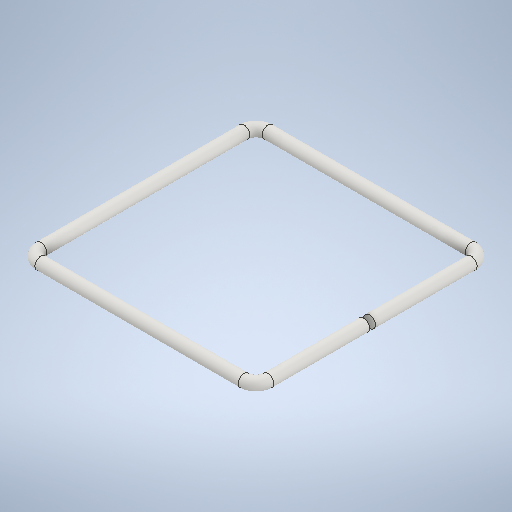
# Autodesk Inventor part: Ring_Of_Rebar
Saved by Autodesk Inventor 2025.1 (Build 291241020, 241B)
## iProperties
Created: 2024-09-07
Part Number: Ring_Of_Rebar
Material: Steel
Document SubType Name: Modeling
Designer: Tom
Density: 7.85 g/cm^3
Appearance: Steel
Author: Tom
Autodesk Inventor part; units mm, degrees
ref_plane "YZ Plane" through (0, 0, 0) normal (1, 0, 0) x (0, 1, 0)
ref_plane "XZ Plane" through (0, 0, 0) normal (0, 1, 0) x (-1, 0, 0)
ref_plane "XY Plane" through (0, 0, 0) normal (0, 0, 1) x (1, 0, 0)
sketch "Sketch1" plane through (0, 0, 0) normal (0, 0, 1) x (1, 0, 0)
  circle A0 centre (0, 0) radius 6.35
  dimension "d0" = 12.7
  constraints: 1 centre point, 1 coincident
  measures "d0" diameter of A0
sketch "Sketch2" plane through (0, 0, 0) normal (0, 1, 0) x (-1, 0, 0)
  line L0 (0, 0) -> (0, -107.95)
  line L1 (12.7, -120.65) -> (228.6, -120.65)
  line L2 (241.3, -107.95) -> (241.3, 107.95)
  line L3 (228.6, 120.65) -> (12.7, 120.65)
  line L4 (0, 107.95) -> (0, 6.35)
  arc A0 (0, -107.95) -> (12.7, -120.65) centre (12.7, -107.95) ccw
  arc A1 (228.6, -120.65) -> (241.3, -107.95) centre (228.6, -107.95) ccw
  arc A2 (241.3, 107.95) -> (228.6, 120.65) centre (228.6, 107.95) ccw
  arc A3 (12.7, 120.65) -> (0, 107.95) centre (12.7, 107.95) ccw
  point P0 (0, -120.65)
  point P1 (241.3, -120.65)
  point P2 (241.3, 120.65)
  point P3 (0, 120.65)
  dimension "d1" = 6.35
  dimension "d2" = 120.65
  dimension "d3" = 241.3
  dimension "d4" = 241.3
  dimension "d8" = 12.7
  constraints: 10 end point, 10 point on line, 8 point on circle, 8 tangent, 4 centre point, 3 equal radius, 2 perpendicular, 1 parallel, 1 vertical
  measures "d1" distance of L4.end L0.start
  measures "d2" distance of L0.start point (0, -120.65)
  measures "d3" distance of point (0, -120.65) point (241.3, -120.65)
  measures "d4" distance of point (241.3, -120.65) point (241.3, 120.65)
  measures "d8" radius of A0
sweep "Sweep1" add profiles "Sketch1" path "Sketch2"
body "Solid1"
